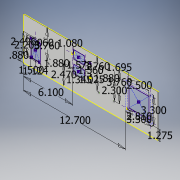
# Autodesk Inventor part: PDU_chassis_back
Saved by Autodesk Inventor 2017 (Build 210142000, 142)
## iProperties
Created: 2017-02-14
Part Number: PDU_chassis_back
Material: Generic
Document SubType Name: Modeling
Designer: Zara
Density: 1 g/cm^3
Appearance: Default
Author: Zara
Autodesk Inventor part; units mm, degrees
ref_plane "YZ Plane" through (0, 0, 0) normal (1, 0, 0) x (0, 1, 0)
ref_plane "XZ Plane" through (0, 0, 0) normal (0, 1, 0) x (-1, 0, 0)
ref_plane "XY Plane" through (0, 0, 0) normal (0, 0, 1) x (1, 0, 0)
sketch "Sketch1" plane through (0, 0, 0) normal (0, 0, 1) x (1, 0, 0)
  line L0 (-212.471, -66.294) -> (212.471, -66.294)
  line L1 (212.471, -66.294) -> (212.471, 66.294)
  line L2 (212.471, 66.294) -> (-212.471, 66.294)
  line L3 (-212.471, 66.294) -> (-212.471, -66.294)
  line L4 (-212.471, -66.294) -> (212.471, 66.294) construction
  line L5 (212.471, -66.294) -> (-212.471, 66.294) construction
  point P0 (0, 0)
  dimension "d0" = 424.942
  dimension "d1" = 132.588
  constraints: 12 end point, 2 midpoint, 2 parallel, 1 horizontal, 1 perpendicular
  measures "d0" distance of L1.end L2.end
  measures "d1" distance of L0.end L1.end
extrude "PDU back" add sketch "Sketch1" along normal blind 1.651
sketch "pwr entry" plane through (0, 0, 1.651) normal (0, 0, 1) x (1, 0, 0)
  line L0 (-187.1218, -40.259) -> (-161.6202, -40.259)
  line L1 (-160.0962, -38.735) -> (-160.0962, 14.224)
  line L2 (-161.6202, 15.748) -> (-187.1218, 15.748)
  line L3 (-188.6458, 14.224) -> (-188.6458, -38.735)
  line L4 (-188.6458, -40.259) -> (-160.0962, 15.748) construction
  line L5 (-160.0962, -40.259) -> (-188.6458, 15.748) construction
  line L6 (-174.371, 19.4437) -> (-174.371, -43.9547) construction
  line L7 (-212.471, 66.294) -> (-212.471, -66.294) projected
  line L8 (-212.471, -66.294) -> (212.471, -66.294) projected
  arc A0 (-160.0962, 14.224) -> (-161.6202, 15.748) centre (-161.6202, 14.224) ccw
  arc A1 (-187.1218, 15.748) -> (-188.6458, 14.224) centre (-187.1218, 14.224) ccw
  arc A2 (-188.6458, -38.735) -> (-187.1218, -40.259) centre (-187.1218, -38.735) ccw
  arc A3 (-161.6202, -40.259) -> (-160.0962, -38.735) centre (-161.6202, -38.735) ccw
  point P0 (0, 0)
  point P1 (-174.371, -12.2555)
  point P2 (-174.371, -12.2555)
  dimension "d4" = 56.007
  dimension "d5" = 28.5496
  dimension "d6" = 63.3984
  dimension "d7" = 38.1
  dimension "d8" = 22.3393
  dimension "d9" = 1.524
  constraints: 14 end point, 8 point on circle, 8 point on line, 8 tangent, 4 centre point, 4 midpoint, 3 equal radius, 2 coincident, 2 parallel, 1 horizontal, 1 perpendicular, 1 vertical
  measures "d4" distance of L5.start L4.end
  measures "d5" distance of L4.start L5.start
  measures "d6" distance of L6.end L6.start
  measures "d7" distance from line of L7 L6.end
  measures "d8" distance from line of point (-174.371, -43.955) L8
  measures "d9" radius of A0
extrude "pwr entry cutout" cut sketch "pwr entry" against normal through all
hole "pwr entry holes" at (-174.371, 19.4437, 1.651) at (-174.371, -43.9547, 1.651) direction (0, 0, -1) diameter 3.4544 end through all
sketch "IEC outlet" plane through (0, 0, 1.651) normal (0, 0, 1) x (1, 0, 0)
  line L0 (-54.61, -16.5735) -> (-20.447, -16.5735)
  line L1 (-20.447, -16.5735) -> (-20.447, 9.4615)
  line L2 (-20.447, 9.4615) -> (-54.61, 9.4615)
  line L3 (-54.61, 9.4615) -> (-54.61, -16.5735)
  line L4 (-54.61, -16.5735) -> (-20.447, 9.4615) construction
  line L5 (-20.447, -16.5735) -> (-54.61, 9.4615) construction
  line L6 (-57.531, -3.556) -> (-17.526, -3.556) construction
  line L7 (-212.471, 66.294) -> (-212.471, -66.294) projected
  line L8 (-212.471, -66.294) -> (212.471, -66.294) projected
  line L9 (-54.61, 23.0505) -> (-20.447, 23.0505)
  line L10 (-20.447, 23.0505) -> (-20.447, 49.0855)
  line L11 (-20.447, 49.0855) -> (-54.61, 49.0855)
  line L12 (-54.61, 49.0855) -> (-54.61, 23.0505)
  line L13 (-54.61, 23.0505) -> (-20.447, 49.0855) construction
  line L14 (-20.447, 23.0505) -> (-54.61, 49.0855) construction
  line L15 (-57.531, 36.068) -> (-17.526, 36.068) construction
  point P0 (0, 0)
  point P1 (-37.5285, -3.556)
  point P2 (-37.5285, -3.556)
  point P3 (0, 39.624)
  point P4 (-37.5285, 36.068)
  point P5 (-37.5285, 36.068)
  dimension "d19" = 26.035
  dimension "d20" = 34.163
  dimension "d22" = 40.005
  dimension "d23" = 154.94
  dimension "d24" = 62.738
  dimension "d27" = 39.624
  constraints: 28 end point, 6 midpoint, 4 coincident, 2 horizontal, 2 parallel, 1 perpendicular, 1 vertical, 18 other
  measures "d19" distance of L0.end L1.end
  measures "d20" distance of L0.start L0.end
  measures "d22" distance of L6.end point (-57.531, -3.556)
  measures "d23" distance from line of L7 L6.start
  measures "d24" distance from line of L6.start L8
  measures "d27" distance of point (0, 0) point (0, 39.624)
hole "IEC holes" at (-17.526, -3.556, 1.651) at (-57.531, -3.556, 1.651) at (-57.531, 36.068, 1.651) at (-17.526, 36.068, 1.651) direction (0, 0, -1) diameter 3.4544 end through all
extrude "IEC cutout" cut sketch "IEC outlet" against normal blind 25.4
sketch "airflow" plane through (0, 0, 1.651) normal (0, 0, 1) x (1, 0, 0)
  line L0 (110.109, -33.909) -> (193.929, -33.909) construction
  line L1 (193.929, -33.909) -> (193.929, 49.911) construction
  line L2 (193.929, 49.911) -> (110.109, 49.911) construction
  line L3 (110.109, 49.911) -> (110.109, -33.909) construction
  line L4 (110.109, -33.909) -> (193.929, 49.911) construction
  line L5 (193.929, -33.909) -> (110.109, 49.911) construction
  line L6 (-212.471, 66.294) -> (-212.471, -66.294) projected
  line L7 (-212.471, -66.294) -> (212.471, -66.294) projected
  line L8 (120.269, -23.749) -> (183.769, -23.749)
  line L9 (183.769, -23.749) -> (183.769, 39.751)
  line L10 (183.769, 39.751) -> (120.269, 39.751)
  line L11 (120.269, 39.751) -> (120.269, -23.749)
  line L12 (120.269, -23.749) -> (183.769, 39.751) construction
  line L13 (183.769, -23.749) -> (120.269, 39.751) construction
  line L14 (116.332, -27.686) -> (187.706, -27.686) construction
  line L15 (187.706, -27.686) -> (187.706, 43.688) construction
  line L16 (187.706, 43.688) -> (116.332, 43.688) construction
  line L17 (116.332, 43.688) -> (116.332, -27.686) construction
  line L18 (116.332, -27.686) -> (187.706, 43.688) construction
  line L19 (187.706, -27.686) -> (116.332, 43.688) construction
  point P0 (0, 0)
  point P1 (152.019, 8.001)
  dimension "d43" = 83.82
  dimension "d44" = 83.82
  dimension "d45" = 322.58
  dimension "d46" = 32.385
  dimension "d47" = 63.5
  dimension "d48" = 71.374
  constraints: 36 end point, 6 midpoint, 6 parallel, 4 point on line, 3 coincident, 3 horizontal, 3 perpendicular
  measures "d43" distance of L0.start L0.end
  measures "d44" distance of L0.end L1.end
  measures "d45" distance between parallel lines of L6 L3
  measures "d46" distance between parallel lines of L0 L7
  measures "d47" distance of L9.end L10.end
  measures "d48" distance of L14.start L14.end
hole "airflow holes" at (187.706, 43.688, 1.651) at (116.332, 43.688, 1.651) at (116.332, -27.686, 1.651) at (187.706, -27.686, 1.651) direction (0, 0, -1) diameter 4.4958 end through all
extrude "airflow cutout" cut sketch "airflow" against normal through all
fillet "IEC fillet 1" radius 4.9784 4 edges at (-54.61, 49.0855, 0.8255) (-20.447, 49.0855, 0.8255) (-20.447, 23.0505, 0.8255) (-54.61, 23.0505, 0.8255)
fillet "IEC fillet 2" radius 4.9784 4 edges at (-54.61, 9.4615, 0.8255) (-54.61, -16.5735, 0.8255) (-20.447, 9.4615, 0.8255) (-20.447, -16.5735, 0.8255)
sketch "Sketch5" plane through (0, 0, 0) normal (0, 0, -1) x (-1, 0, 0)
  circle A0 centre (-116.332, 43.688) radius 2.2479 construction
  circle A1 centre (-116.332, -27.686) radius 2.2479 construction
  circle A2 centre (-116.332, -27.686) radius 2.2479 construction
  line L0 (-116.332, 43.688) -> (-116.332, -27.686) construction
  circle A3 centre (17.526, 36.068) radius 1.7272 construction
  circle A4 centre (17.526, -3.556) radius 1.7272 construction
  line L1 (17.526, 36.068) -> (17.526, -3.556) construction
  line L2 (-73.279, 29.21) -> (-25.527, 29.21) construction
  line L3 (84.963, -29.21) -> (132.715, -29.21) construction
  circle A5 centre (57.531, 36.068) radius 1.7272 construction
  line L4 (-25.5336, -29.21) -> (147.9977, -29.21) construction
  line L5 (84.9503, 23.1654) -> (84.9503, -54.0444) construction
  line L6 (-212.471, 66.294) -> (212.471, 66.294) projected
  point P0 (0, 0)
  point P1 (0, 0)
  point P2 (-73.279, -29.21)
  dimension "d60" = 58.42
  dimension "d61" = 47.752
  dimension "d62" = 27.432
  dimension "d63" = 47.752
  dimension "d64" = 43.053
  dimension "d73" = 95.504
  dimension "d74" = 95.504
  dimension "d75" = 95.504
  constraints: 12 end point, 3 horizontal, 3 vertical
  measures "d60" distance of L2.start point (-73.279, -29.21)
  measures "d61" distance of L2.start L2.end
  measures "d62" horizontal distance of A5.centre L3.start
  measures "d63" distance of L3.end L3.start
  measures "d64" distance from line of L0 L2.start
  measures "d73" distance from line of L6 point (-73.279, -29.21)
  measures "d74" distance from line of L6 L4.start
  measures "d75" distance from line of L3.end L6
sketch "Sketch6" plane through (0, 0, 1.651) normal (0, 0, 1) x (1, 0, 0)
  line L0 (73.279, -29.21) -> (-149.3427, -29.21) construction
  line L1 (-132.7023, 25.4917) -> (-132.7023, -42.1158) construction
  point P0 (0, 0)
  point P1 (73.279, 29.21)
  point P2 (25.527, 29.21)
  point P3 (25.5336, -29.21)
  point P4 (-84.963, -29.21)
  point P5 (-132.715, -29.21)
  constraints: 4 end point, 1 horizontal, 1 vertical
hole "solid state relay holes" at (-132.715, -29.21, 1.651) at (-84.963, -29.21, 1.651) at (25.527, 29.21, 1.651) at (73.279, 29.21, 1.651) at (25.5336, -29.21, 1.651) at (73.279, -29.21, 1.651) direction (0, 0, -1) diameter 4.4958 end through all clearance for "Flat Head Machine Screw (82)" size "#8" standard "Ansi Unified Screw Threads"
body "Solid1"
